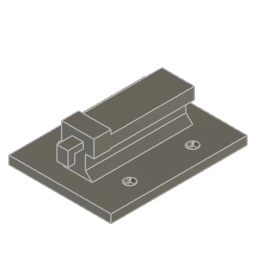
Clip Drone (Autodesk Fusion 360 design; units mm, degrees)
Autodesk Fusion 360 part; units mm, degrees
sketch "Esquisse1" plane through (0, 0, 0) normal (0, 0, 1) x (1, 0, 0)
  line L0 (-30, 40) -> (30, 40)
  line L1 (30, 40) -> (30, -40)
  line L2 (30, -40) -> (-30, -40)
  line L3 (-30, -40) -> (-30, 40)
  line L4 (-30, 40) -> (30, -40) construction
  line L5 (30, 40) -> (-30, -40) construction
  dimension "d1" = 60
  dimension "d2" = 80
  constraint horizontal L0
  constraint perpendicular L0 L1
  constraint parallel L0 L2
  constraint parallel L1 L3
  constraint coincident L4 origin
  constraint coincident L5 origin
  measures "d1" distance of L0.start L0.end
  measures "d2" distance of L0.start L2.end
extrude "Extrusion1" add sketch "Esquisse1" along normal blind 5
sketch "Esquisse2" plane through (0, 0, 5) normal (0, 0, 1) x (-1, 0, 0)
  line L0 (30, 40) -> (-30, 40)
  line L1 (-30, 40) -> (-30, -40)
  line L2 (-30, -40) -> (30, -40)
  line L3 (30, -40) -> (30, 40)
  line L4 (4.5, -29.5) -> (-4.5, -29.5)
  line L5 (-4.5, -29.5) -> (-4.5, 29.5)
  line L6 (-4.5, 29.5) -> (4.5, 29.5)
  line L7 (4.5, 29.5) -> (4.5, -29.5)
  line L8 (4.5, -29.5) -> (-4.5, 29.5) construction
  line L9 (-4.5, -29.5) -> (4.5, 29.5) construction
  dimension "d5" = 59
  dimension "d6" = 9
  constraint horizontal L4
  constraint perpendicular L4 L5
  constraint parallel L4 L6
  constraint parallel L5 L7
  constraint coincident L8 origin
  constraint coincident L9 origin
  measures "d5" distance of L4.end L5.end
  measures "d6" distance of L4.start L4.end
extrude "Extrusion2" add sketch "Esquisse2" along normal blind 17 contours L4 L5 L6 L7
sketch "Esquisse3" plane through (0, 0, 22) normal (0, 0, 1) x (-1, 0, 0)
  line L0 (4.5, 29.5) -> (-4.5, 29.5)
  line L1 (-4.5, 29.5) -> (-4.5, -29.5)
  line L2 (-4.5, -29.5) -> (4.5, -29.5)
  line L3 (4.5, -29.5) -> (4.5, 29.5)
  line L4 (9.5, -29.5) -> (-9.5, -29.5)
  line L5 (-9.5, -29.5) -> (-9.5, 29.5)
  line L6 (-9.5, 29.5) -> (9.5, 29.5)
  line L7 (9.5, 29.5) -> (9.5, -29.5)
  line L8 (9.5, -29.5) -> (-9.5, 29.5) construction
  line L9 (-9.5, -29.5) -> (9.5, 29.5) construction
  dimension "d9" = 59
  dimension "d10" = 19
  constraint horizontal L4
  constraint perpendicular L4 L5
  constraint parallel L4 L6
  constraint parallel L5 L7
  constraint coincident L8 origin
  constraint coincident L9 origin
  measures "d9" distance of L4.end L5.end
  measures "d10" distance of L4.start L4.end
extrude "Extrusion3" add sketch "Esquisse3" along normal blind 3
sketch "Esquisse4" plane through (0, 0, 25) normal (0, 0, 1) x (-1, 0, 0)
  line L0 (9.5, 29.5) -> (-9.5, 29.5)
  line L1 (-9.5, 29.5) -> (-9.5, -29.5)
  line L2 (-9.5, -29.5) -> (9.5, -29.5)
  line L3 (9.5, -29.5) -> (9.5, 29.5)
  line L4 (-9.5, 29.5) -> (9.5, 29.5)
  line L5 (9.5, 29.5) -> (9.5, 19.5)
  line L6 (9.5, 19.5) -> (-9.5, 19.5)
  line L7 (-9.5, 19.5) -> (-9.5, 29.5)
  dimension "d13" = 10
  constraint horizontal L4
  constraint vertical L5
  constraint horizontal L6
  constraint vertical L7
  constraint coincident L3 L5.end
  constraint coincident L0.end L1.start
  measures "d13" distance of L0.start L5.end
extrude "Extrusion4" add sketch "Esquisse4" along normal blind 10 from surface at -7.5 contours L0 L1 L3 L4 L5 L6 L7
chamfer "Chanfrein5" distance 4 angle 45 1 edges at (4.5, 0, 5)
chamfer "Chanfrein6" distance 4 angle 45 1 edges at (-4.5, 0, 5)
sketch "Esquisse10" plane through (0, -29.5, 0) normal (0, -1, 0) x (1, 0, 0)
  line L0 (9.5, 17.5) -> (9.5, 27.5)
  line L1 (-9.5, 27.5) -> (-9.5, 17.5)
  line L2 (-4.5, 17.5) -> (-4.5, 9)
  line L3 (-4.5, 9) -> (-8.5, 5)
  line L4 (-8.5, 5) -> (8.5, 5)
  line L5 (8.5, 5) -> (4.5, 9)
  line L6 (4.5, 9) -> (4.5, 17.5)
  line L7 (0, 25) -> (0, 23)
  line L8 (0, 23) -> (-3.25, 23)
  line L9 (-3.25, 23) -> (3.25, 23)
  line L10 (3.25, 23) -> (3.25, 14.5)
  line L11 (3.25, 14.5) -> (-3.25, 14.5)
  line L12 (-3.25, 14.5) -> (-3.25, 23)
  line L13 (-3.25, 23) -> (3.25, 23)
  line L14 (3.25, 23) -> (3.25, 19.5)
  line L15 (3.25, 19.5) -> (-3.25, 19.5)
  line L16 (-3.25, 19.5) -> (-3.25, 23)
  line L17 (4.5, 17.5) -> (9.5, 17.5)
  line L18 (9.5, 27.5) -> (-9.5, 27.5)
  line L19 (-9.5, 27.5) -> (9.5, 27.5)
  line L20 (-9.5, 17.5) -> (-4.5, 17.5)
  point P0 (0, 25)
  point P1 (0, 23)
  dimension "d33" = 6.5
  dimension "d34" = 3.5
  dimension "d35" = 8.5
  dimension "d46" = 4.5
  constraint coincident P0 L7.start
  constraint perpendicular L7 L8
  constraint horizontal L9
  constraint vertical L10
  constraint horizontal L11
  constraint vertical L12
  constraint horizontal L13
  constraint vertical L14
  constraint horizontal L15
  constraint vertical L16
  constraint coincident L10 L14.end
  constraint midpoint L9 P1
  constraint coincident P1 L7.end
  constraint coincident L1.start L18.end
  constraint coincident L0.end L18.start
  measures "d33" distance of L8.end L9.end
  measures "d34" distance of L8.end L15.end
  measures "d35" distance of L8.end L11.end
  measures "d46" distance of L9 L19
extrude "Extrusion9" add sketch "Esquisse10" along normal blind 6 contours L8 L9 L10 L12 L13 L14 L15 L16
extrude "Extrusion10" add sketch "Esquisse10" along normal blind 4 from surface at 5 contours L8 L9 L10 L12 L13 L14 L15 L16 | L10 L11 L12 L15
extrude "Extrusion11" add 2 faces at (7.8333, 13.1667, 22) (-7.8333, 13.1667, 22) along direction (0, 0, -1) blind 4
sketch "Esquisse11" plane through (0, 0, 5) normal (0, 0, 1) x (-1, 0, 0)
  line L0 (8.5, -29.5) -> (-8.5, -29.5)
  line L1 (-8.5, -29.5) -> (-8.5, 29.5)
  line L2 (-8.5, 29.5) -> (8.5, 29.5)
  line L3 (8.5, 29.5) -> (8.5, -29.5)
  line L4 (30, 40) -> (-30, 40)
  line L5 (-30, 40) -> (-30, -40)
  line L6 (-30, -40) -> (30, -40)
  line L7 (30, -40) -> (30, 40)
  circle A0 centre (19, -19) radius 1.55
  circle A1 centre (19, 18) radius 1.55
  circle A2 centre (-19, -19) radius 1.55
  circle A3 centre (-19, 18) radius 1.55
  dimension "d47" = 3.1
  dimension "d48" = 3.1
  dimension "d49" = 3.1
  dimension "d50" = 3.1
  dimension "d51" = 37
  dimension "d52" = 37
  dimension "d53" = 11
  dimension "d54" = 11
  dimension "d55" = 11
  dimension "d56" = 11
  dimension "d57" = 22
  dimension "d58" = 22
  measures "d47" diameter of A3
  measures "d48" diameter of A2
  measures "d49" diameter of A0
  measures "d50" diameter of A1
  measures "d51" vertical distance of A0.centre A1.centre
  measures "d52" distance of A2.centre A3.centre
  measures "d53" distance of L7 A1.centre
  measures "d54" distance of L7 A0.centre
  measures "d55" distance of L5 A3.centre
  measures "d56" distance of L5 A2.centre
  measures "d57" distance of L4 A1.centre
  measures "d58" distance of L4 A3.centre
extrude "Extrusion12" cut sketch "Esquisse11" against normal blind 10 contours A0 | A1 | A2 | A3
chamfer "Chanfrein7" distance 1.5 angle 45 4 edges at (-17.5549, 18.4395, 5) (-17.5549, -18.5605, 5) (20.4451, 18.4395, 5) (20.4451, -18.5605, 5)
